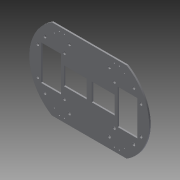
# Autodesk Inventor part: base
Saved by Autodesk Inventor 2015 (Build 190159000, 159)
## iProperties
Created: 2014-09-21
Part Number: base
Material: Générique
Document SubType Name: Modeling
Designer: astralien3000
Density: 1 g/cm^3
Appearance: Par défaut
Author: astralien3000
Autodesk Inventor part; units mm, degrees
ref_plane "YZ Plane" through (0, 0, 0) normal (1, 0, 0) x (0, 1, 0)
ref_plane "XZ Plane" through (0, 0, 0) normal (0, 1, 0) x (-1, 0, 0)
ref_plane "XY Plane" through (0, 0, 0) normal (0, 0, 1) x (1, 0, 0)
sketch "Esquisse1" plane through (0, 0, 0) normal (0, 1, 0) x (-1, 0, 0)
  circle A0 centre (0, 0) radius 25 construction
  line L0 (-25, 0) -> (25, 0) construction
  arc A1 (-75, -80.7775) -> (-75, 80.7775) centre (-25, 0) ccw construction
  arc A2 (75, 80.7775) -> (75, -80.7775) centre (25, 0) ccw construction
  line L1 (0, 25) -> (0, 0) construction
  line L2 (-75, 80.7775) -> (75, 80.7775)
  line L3 (-75, -80.7775) -> (75, -80.7775)
  arc A3 (75, -80.7775) -> (75, 80.7775) centre (25, 0) ccw
  arc A4 (-75, 80.7775) -> (-75, -80.7775) centre (-25, 0) ccw
  dimension "d0" = 50
  dimension "d1" = 190
  dimension "d2" = 150
  constraints: 11 point on circle, 8 end point, 5 centre point, 3 coincident, 2 perpendicular, 1 horizontal, 1 midpoint, 2 other
  measures "d0" diameter of A0
  measures "d1" diameter of A1
  measures "d2" distance of L2.start L2.end
extrude "Extrusion1" add sketch "Esquisse1" along normal blind 3
sketch "Esquisse4" plane through (0, 0, 0) normal (0, -1, 0) x (1, 0, 0)
  line L0 (-50, 40) -> (50, 40) construction
  line L1 (50, 40) -> (50, -40) construction
  line L2 (50, -40) -> (-50, -40) construction
  line L3 (-50, -40) -> (-50, 40) construction
  circle A0 centre (-50, 40) radius 3
  circle A1 centre (50, 40) radius 3
  circle A2 centre (50, -40) radius 3
  circle A3 centre (-50, -40) radius 3
  line L4 (75, 80.7775) -> (-75, 80.7775) projected
  point P0 (0, 0)
  dimension "d15" = 80
  dimension "d16" = 100
  dimension "d17" = 50
  dimension "d18" = 40
  dimension "d19" = 6
  dimension "d20" = 6
  dimension "d21" = 6
  dimension "d22" = 6
  dimension "d25" = 40.7775
  constraints: 8 end point, 4 centre point, 4 coincident, 2 parallel, 1 horizontal, 1 perpendicular
  measures "d15" distance of L0.end L1.end
  measures "d16" distance of L0.start L0.end
  measures "d17" distance from line of L1 point (0, 0)
  measures "d18" distance from line of L2 point (0, 0)
  measures "d19" diameter of A0
  measures "d20" diameter of A1
  measures "d21" diameter of A2
  measures "d22" diameter of A3
  measures "d25" distance between parallel lines of L4 L0
extrude "Extrusion4" cut sketch "Esquisse4" against normal through all
sketch "Esquisse5" plane through (0, 0, 0) normal (0, -1, 0) x (1, 0, 0)
  arc A0 (-75, 80.7775) -> (-75, -80.7775) centre (-25, 0) ccw projected
  line L0 (-96.5, 35) -> (-70.8, 35)
  line L1 (-70.8, 35) -> (-70.8, -35)
  line L2 (-70.8, -35) -> (-96.5, -35)
  line L3 (-96.5, -35) -> (-96.5, 35)
  line L4 (-70.8, 35) -> (-66.8, 35)
  line L5 (-66.8, 35) -> (-66.8, -35)
  line L6 (-66.8, -35) -> (-70.8, -35)
  line L7 (-70.8, -35) -> (-70.8, 35)
  line L8 (-66.8, 35) -> (-56.8, 35)
  line L9 (-56.8, 35) -> (-56.8, -35)
  line L10 (-56.8, -35) -> (-66.8, -35)
  line L11 (-66.8, -35) -> (-66.8, 35)
  line L12 (0, 0) -> (-120, 0) construction
  dimension "d26" = 4
  dimension "d27" = 70
  dimension "d28" = 35
  dimension "d29" = 25.7
  dimension "d30" = 10
  dimension "d31" = 23.5
  dimension "d80" = 56.8
  constraints: 26 end point, 6 parallel, 3 horizontal, 3 perpendicular, 2 collinear, 1 point on circle
  measures "d26" distance between parallel lines of L5 L1
  measures "d27" distance between parallel lines of L10 L8
  measures "d28" vertical distance of L9.end L12.start
  measures "d29" distance between parallel lines of L1 L3
  measures "d30" distance between parallel lines of L5 L9
  measures "d31" distance from line of L3 L12.end
  measures "d80" distance from line of L12.start L9
extrude "Extrusion5" cut sketch "Esquisse5" against normal through all
mirror "Symétrie1" about plane through (0, 0, 0) normal (1, 0, 0) of "Extrusion5"
sketch "Esquisse8" plane through (0, 0, 0) normal (0, -1, 0) x (1, 0, 0)
  line L0 (96.5, 35) -> (96.5, -35) projected
  line L1 (82, 42) -> (96, 42)
  line L2 (96, 42) -> (96, -42)
  line L3 (96, -42) -> (82, -42)
  line L4 (82, -42) -> (82, 42)
  line L5 (96, 21.5) -> (108.5, 21.5)
  line L6 (108.5, 21.5) -> (108.5, -21.5)
  line L7 (108.5, -21.5) -> (96, -21.5)
  line L8 (96, -21.5) -> (96, 21.5)
  line L9 (82, -14.7) -> (76.3, -14.7)
  line L10 (76.3, -14.7) -> (76.3, 14.7)
  line L11 (76.3, 14.7) -> (82, 14.7)
  line L12 (82, 14.7) -> (82, -14.7)
  line L13 (82, 14.7) -> (72, 14.7)
  line L14 (72, 14.7) -> (72, 24.7)
  line L15 (72, 24.7) -> (82, 24.7)
  line L16 (82, 24.7) -> (82, 14.7)
  line L17 (96, 21.5) -> (110.5, 21.5)
  line L18 (110.5, 21.5) -> (110.5, 35.5)
  line L19 (110.5, 35.5) -> (96, 35.5)
  line L20 (96, 35.5) -> (96, 21.5)
  line L21 (96, 42) -> (82, 42)
  line L22 (82, 42) -> (82, 56)
  line L23 (82, 56) -> (96, 56)
  line L24 (96, 56) -> (96, 42)
  line L25 (72, 24.7) -> (82, 14.7) construction
  line L26 (82, 24.7) -> (72, 14.7) construction
  line L27 (110.5, 21.5) -> (96, 35.5) construction
  line L28 (96, 21.5) -> (110.5, 35.5) construction
  line L29 (82, 56) -> (96, 42) construction
  line L30 (82, 42) -> (96, 56) construction
  circle A0 centre (89, 49) radius 3
  circle A1 centre (77, 19.7) radius 3
  circle A2 centre (103.25, 28.5) radius 3
  arc A3 (75, -80.7775) -> (75, 80.7775) centre (25, 0) ccw projected
  line L31 (108.5, 21.5) -> (115, 21.5)
  line L32 (115, 21.5) -> (115, -21.5)
  line L33 (115, -21.5) -> (108.5, -21.5)
  line L34 (108.5, -21.5) -> (108.5, 21.5)
  line L35 (0, 0) -> (120, 0)
  dimension "d59" = 84
  dimension "d60" = 14
  dimension "d61" = 29.4
  dimension "d62" = 5.7
  dimension "d63" = 12.5
  dimension "d64" = 43
  dimension "d65" = 42
  dimension "d66" = 14.7
  dimension "d67" = 21.5
  dimension "d68" = 14
  dimension "d69" = 14
  dimension "d70" = 14
  dimension "d71" = 10
  dimension "d72" = 10
  dimension "d73" = 6
  dimension "d74" = 6
  dimension "d75" = 6
  dimension "d78" = 6.5
  dimension "d79" = 5
  constraints: 70 end point, 14 parallel, 8 perpendicular, 7 horizontal, 3 centre point, 3 midpoint, 3 point on line, 2 collinear, 1 point on circle
  measures "d59" distance of L3.end L1.start
  measures "d60" distance of L1.start L1.end
  measures "d61" distance of L9.end L10.end
  measures "d62" distance of L10.end L11.end
  measures "d63" distance of L5.start L5.end
  measures "d64" distance of L5.end L6.end
  measures "d65" distance from line of L35.start L1
  measures "d66" distance from line of L35.start L11
  measures "d67" distance from line of L35.start L5
  measures "d68" distance between parallel lines of L1 L23
  measures "d69" distance between parallel lines of L0 L18
  measures "d70" distance of L17.end L18.end
  measures "d71" distance between parallel lines of L13 L15
  measures "d72" distance of L14.end L15.end
  measures "d73" diameter of A1
  measures "d74" diameter of A0
  measures "d75" diameter of A2
  measures "d78" distance between parallel lines of L6 L32
  measures "d79" distance from line of L32 L35.end
extrude "Extrusion6" cut sketch "Esquisse8" against normal through all contours A0 | A1 | A2
mirror "Symétrie2" about plane through (0, 0, 0) normal (0, 0, 1) of "Extrusion6"
mirror "Symétrie3" about plane through (0, 0, 0) normal (1, 0, 0) of "Extrusion6", "Symétrie2"
sketch "Esquisse9" plane through (0, 0, 0) normal (0, -1, 0) x (1, 0, 0)
  line L0 (56.8, -35) -> (56.8, 35) projected
  line L1 (5, 18) -> (50.8, 18)
  line L2 (50.8, 18) -> (50.8, -18)
  line L3 (50.8, -18) -> (5, -18)
  line L4 (5, -18) -> (5, 18)
  point P0 (0, 0)
  dimension "d81" = 36
  dimension "d82" = 18
  dimension "d83" = 6
  dimension "d84" = 5
  constraints: 8 end point, 2 parallel, 1 horizontal, 1 perpendicular
  measures "d81" distance between parallel lines of L3 L1
  measures "d82" distance from line of point (0, 0) L1
  measures "d83" distance between parallel lines of L0 L2
  measures "d84" distance from line of point (0, 0) L4
extrude "Extrusion7" cut sketch "Esquisse9" against normal through all
mirror "Symétrie4" about plane through (0, 0, 0) normal (1, 0, 0) of "Extrusion7"
sketch "Esquisse10" plane through (0, 0, 0) normal (0, -1, 0) x (1, 0, 0)
  circle A0 centre (70, 65) radius 1.25
  point P0 (0, 0)
  dimension "d87" = 65
  dimension "d88" = 70
  dimension "d89" = 2.5
  constraints: 1 centre point
  measures "d87" vertical distance of A0.centre point (0, 0)
  measures "d88" horizontal distance of point (0, 0) A0.centre
  measures "d89" diameter of A0
extrude "Extrusion8" cut sketch "Esquisse10" against normal through all
mirror "Symétrie5" about plane through (0, 0, 0) normal (1, 0, 0) of "Extrusion8"
mirror "Symétrie6" about plane through (0, 0, 0) normal (0, 0, 1) of "Extrusion8", "Symétrie5"
sketch "Esquisse11" plane through (0, 0, 0) normal (0, -1, 0) x (1, 0, 0)
  line L0 (-65, 79.7775) -> (-45, 79.7775)
  line L1 (-45, 79.7775) -> (-45, 69.7775)
  line L2 (-45, 69.7775) -> (-65, 69.7775)
  line L3 (-65, 69.7775) -> (-65, 79.7775)
  line L4 (-75, 80.7775) -> (75, 80.7775) projected
  circle A0 centre (-70, 65) radius 1.25 projected
  circle A1 centre (-70, 65) radius 10
  circle A2 centre (-60, 72.7775) radius 1.5
  circle A3 centre (-50, 72.7775) radius 1.5
  point P0 (0, 0)
  dimension "d92" = 10
  dimension "d93" = 20
  dimension "d94" = 1
  dimension "d95" = 5
  dimension "d96" = 20
  dimension "d97" = 3
  dimension "d98" = 3
  dimension "d99" = 3
  dimension "d100" = 3
  dimension "d101" = 5
  dimension "d102" = 5
  constraints: 8 end point, 3 centre point, 2 parallel, 1 coincident, 1 horizontal, 1 perpendicular
  measures "d92" distance of L2.end L0.start
  measures "d93" distance of L0.start L0.end
  measures "d94" distance between parallel lines of L4 L0
  measures "d95" distance from line of A0.centre L3
  measures "d96" diameter of A1
  measures "d97" diameter of A2
  measures "d98" diameter of A3
  measures "d99" distance from line of L2 A3.centre
  measures "d100" distance from line of L2 A2.centre
  measures "d101" distance from line of L1 A3.centre
  measures "d102" distance from line of L3 A2.centre
extrude "Extrusion9" cut sketch "Esquisse11" against normal through all contours A2 | A3
mirror "Symétrie7" about plane through (0, 0, 0) normal (1, 0, 0) of "Extrusion9"
mirror "Symétrie8" about plane through (0, 0, 0) normal (0, 0, 1) of "Extrusion9", "Symétrie7"
sketch "Esquisse12" plane through (0, 0, 0) normal (0, -1, 0) x (1, 0, 0)
  line L0 (-40, 60) -> (40, 60) construction
  line L1 (40, 60) -> (40, -60) construction
  line L2 (40, -60) -> (-40, -60) construction
  line L3 (-40, -60) -> (-40, 60) construction
  circle A0 centre (-40, 60) radius 3
  circle A1 centre (40, 60) radius 3
  circle A2 centre (-40, -60) radius 3
  circle A3 centre (40, -60) radius 3
  point P0 (0, 0)
  dimension "d105" = 80
  dimension "d106" = 120
  dimension "d107" = 60
  dimension "d108" = 40
  dimension "d109" = 6
  dimension "d110" = 6
  dimension "d111" = 6
  dimension "d112" = 6
  constraints: 8 end point, 4 centre point, 4 coincident, 2 parallel, 1 horizontal, 1 perpendicular
  measures "d105" distance of L0.start L0.end
  measures "d106" distance of L0.end L1.end
  measures "d107" distance from line of point (0, 0) L0
  measures "d108" distance from line of L1 point (0, 0)
  measures "d109" diameter of A0
  measures "d110" diameter of A1
  measures "d111" diameter of A3
  measures "d112" diameter of A2
extrude "Extrusion10" cut sketch "Esquisse12" against normal through all
equation "\"d17\" = 0.5 * d16"
equation "\"d18\" = 0.5 * d15"
equation "\"d20\" = d19"
equation "\"d21\" = d19"
equation "\"d22\" = d19"
equation "\"d28\" = 0.5 * d27"
equation "\"d65\" = 0.5 * d59"
equation "\"d66\" = 0.5 * d61"
equation "\"d67\" = 0.5 * d64"
equation "\"d68\" = d60"
equation "\"d70\" = d69"
equation "\"d82\" = 0.5 * d81"
